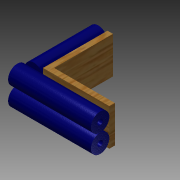
# Autodesk Inventor part: Corner Bumper
Saved by Autodesk Inventor 2015 (Build 190159000, 159)
## iProperties
Created: 2016-01-19
Part Number: Corner Bumper
Material: Generic
Document SubType Name: Modeling
Designer: sethbattis
Density: 1 g/cm^3
Appearance: Default
Author: sethbattis
Autodesk Inventor part; units mm, degrees
ref_plane "YZ Plane" through (0, 0, 0) normal (1, 0, 0) x (0, 1, 0)
ref_plane "XZ Plane" through (0, 0, 0) normal (0, 1, 0) x (-1, 0, 0)
ref_plane "XY Plane" through (0, 0, 0) normal (0, 0, 1) x (1, 0, 0)
sketch "Sketch1" plane through (0, 0, 0) normal (0, 1, 0) x (-1, 0, 0)
  line L0 (0, 0) -> (19.05, 0)
  line L1 (19.05, 0) -> (19.05, -203.2)
  line L2 (19.05, -203.2) -> (0, -203.2)
  line L3 (0, -203.2) -> (0, 0)
  line L4 (19.05, 0) -> (-209.55, 0)
  line L5 (-209.55, 0) -> (-209.55, 19.05)
  line L6 (-209.55, 19.05) -> (19.05, 19.05)
  line L7 (19.05, 19.05) -> (19.05, 0)
  dimension "d0" = 19.05
  dimension "d1" = 203.2
  dimension "d2" = 228.6
  constraints: 16 end point, 4 parallel, 3 perpendicular, 2 horizontal
  measures "d0" distance of L1.end L2.end
  measures "d1" distance of L0.end L1.end
  measures "d2" distance of L5.end L6.end
extrude "Extrusion1" add sketch "Sketch1" along normal blind 127
sketch "Sketch2" plane through (209.55, 0, 19.05) normal (1, 0, 0) x (0, 0, -1)
  circle A0 centre (-31.75, 95.25) radius 31.75
  circle A1 centre (-31.75, 95.25) radius 9.525
  line L0 (0, 0) -> (0, 127) projected
  line L1 (222.25, 127) -> (0, 127) projected
  line L2 (21.2181, 127) -> (-100.8948, 127) construction
  circle A2 centre (-31.75, 31.75) radius 31.75
  circle A3 centre (-31.75, 31.75) radius 9.525
  point P0 (19.05, 0)
  dimension "d6" = 63.5
  dimension "d7" = 19.05
  constraints: 4 centre point, 4 tangent, 2 coincident, 2 end point, 2 equal radius, 1 horizontal, 1 point on line
  measures "d6" diameter of A0
  measures "d7" diameter of A1
extrude "Extrusion2" add sketch "Sketch2" against normal blind 285.75 contours A0 | A2
sketch "Sketch3" plane through (0, 0, -203.2) normal (0, 0, -1) x (-1, 0, 0)
  circle A0 centre (50.8, 95.25) radius 31.75
  line L0 (-209.55, 127) -> (76.2, 127) projected
  line L1 (19.05, 0) -> (19.05, 127) projected
  line L2 (-209.55, 63.5) -> (76.2, 63.5) projected
  circle A1 centre (50.8, 95.25) radius 9.525
  circle A2 centre (50.8, 29.87) radius 31.75
  circle A3 centre (50.8, 29.87) radius 9.525
  point P0 (0, 0)
  dimension "d10" = 19.05
  constraints: 4 centre point, 4 tangent, 2 coincident, 2 equal radius
  measures "d10" diameter of A1
extrude "Extrusion3" add sketch "Sketch3" against normal blind 222.25 contours A0 | A2
body "Solid1"
